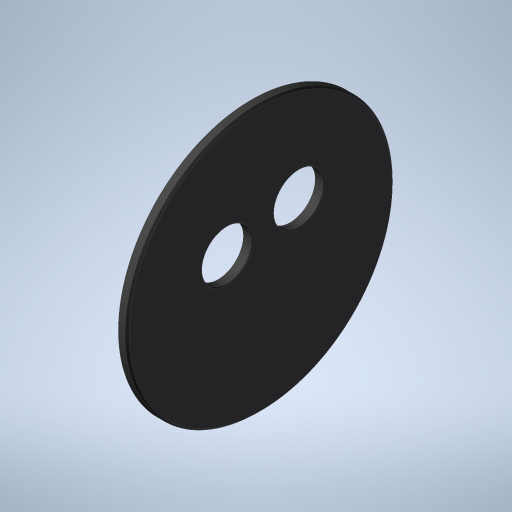
# Autodesk Inventor part: PlateGantryMountSymbolDisc
Saved by Autodesk Inventor 2023 (Build 270158000, 158)
## iProperties
Created: 2026-01-27
Part Number: PlateGantryMountSymbolDisc
Material: Generic
Document SubType Name: Modeling
Designer: DanAr
Density: 1 g/cm^3
Appearance: Default
Author: DanAr
Autodesk Inventor part; units mm, degrees
ref_plane "YZ Plane" through (0, 0, 0) normal (1, 0, 0) x (0, 1, 0)
ref_plane "XZ Plane" through (0, 0, 0) normal (0, 1, 0) x (-1, 0, 0)
ref_plane "XY Plane" through (0, 0, 0) normal (0, 0, 1) x (1, 0, 0)
sketch "Sketch1" plane through (0, 0, 0) normal (1, 0, 0) x (0, 1, 0)
  circle A0 centre (1.9588, 3.377) radius 2.2698
  circle A1 centre (1.9588, 3.377) radius 2.2698
  line L0 (1.9588, 3.377) -> (1.9588, 0)
  line L1 (1.9588, 0) -> (0, 0)
  line L2 (0, 0) -> (0, 3.377)
  line L3 (0, 3.377) -> (1.9588, 3.377)
  circle A2 centre (3.3027, -3.8845) radius 2.2698
  line L4 (0, 0) -> (0, -3.8845)
  line L5 (0, -3.8845) -> (3.3027, -3.8845)
  line L6 (3.3027, -3.8845) -> (3.3027, 0)
  line L7 (3.3027, 0) -> (0, 0)
  circle A3 centre (0, 0) radius 13.5
  dimension "d0" = 4.5396
  dimension "d1" = 3.377
  dimension "d2" = 1.9588
  dimension "d3" = 3.8845
  dimension "d4" = 3.3026
  dimension "d5" = 4.5396
  dimension "d6" = 27
  constraints: 16 end point, 4 centre point, 4 parallel, 2 coincident, 2 perpendicular
  measures "d0" diameter of A0
  measures "d1" distance of L0.start L0.end
  measures "d2" distance of L0.end L1.end
  measures "d3" distance of L5.end L6.end
  measures "d4" distance of L6.end L1.end
  measures "d5" diameter of A2
  measures "d6" diameter of A3
extrude "Extrusion1" add sketch "Sketch1" along normal blind 0.95 contours A0 L0 L1 L2 | L1 L7 L6 A2 L5 L4 | A3
sketch "Sketch2" plane through (0.95, 0, 0) normal (1, 0, 0) x (0, 0, -1)
  circle A0 centre (-3.377, 1.9588) radius 2.2698 projected
  circle A1 centre (-3.377, 1.9588) radius 2.5
  circle A2 centre (3.8845, 3.3027) radius 2.2698 projected
  circle A3 centre (3.8845, 3.3027) radius 2.5
  point P0 (0, 0)
  dimension "d9" = 5
  dimension "d10" = 5
  constraints: 2 centre point, 2 coincident
  measures "d9" diameter of A3
  measures "d10" diameter of A1
extrude "Extrusion2" cut sketch "Sketch2" against normal blind 0.95 contours A0 | A1 | A2 | A3
fillet "Fillet1" radius 0.1 5 edges at (0.95, 1.9588, 5.877) (0.95, 3.3027, -1.3845) (0, 3.3027, -1.3845) (0, 1.9588, 5.877) (0, -13.5, 0)
chamfer "Chamfer1" distance 0.2 angle 45 1 edges at (0.95, -13.5, 0)
body "Solid1"
